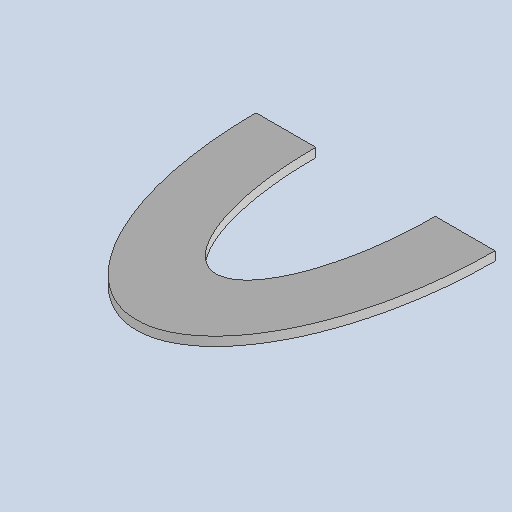
# Autodesk Inventor part: MSC 082 pillar 2
Saved by Autodesk Inventor 2025 (Build 290162010, 162A)
## iProperties
Created: 2024-06-25
Part Number: MSC 082 pillar 2
Material: Stainless Steel
Document SubType Name: Sheet Metal
Designer: admin
Density: 8 g/cm^3
Sheet Metal Rule: AISI304 3mm Die 32
Appearance: Default
Stock Number: Зап. часть
Mass: 80.4248 g
Surface Area: 77.6704 cm^2
Volume: 10.0531 cm^3
Flat Pattern Width: 8 cm
Flat Pattern Length: 8 cm
Flat Pattern Area: 64 cm^2
Sheet Metal Width: 80,000 mm
Sheet Metal Length: 80,000 mm
Sheet Metal Area: 6400,000 mm^2
Author: admin
Autodesk Inventor part; units mm, degrees
ref_plane "YZ Plane" through (0, 0, 0) normal (1, 0, 0) x (0, 1, 0)
ref_plane "XZ Plane" through (0, 0, 0) normal (0, 1, 0) x (-1, 0, 0)
ref_plane "XY Plane" through (0, 0, 0) normal (0, 0, 1) x (1, 0, 0)
sketch "Sketch1" plane through (0, 0, 0) normal (0, 0, 1) x (1, 0, 0)
  ellipse E0 centre (0, 0) end of major axis (0, -80) minor radius 40
  ellipse E1 centre (0, 0) end of major axis (0, -53.3333) minor radius 20
  line L0 (40, 0) -> (-40, 0)
  point P0 (-20, 0)
  point P1 (20, 0)
  dimension "d73" = 80
  dimension "d74" = 40
  dimension "d75" = 20
  dimension "d76" = 53.3333
extrude "Plate1" add sketch "Sketch1" along normal blind 3 contours E0 L0 E1 picked at (-33.0642, -5.3304)
equation "\"d75\" = 0.5 * d74"
equation "\"d76\" = 0.666667 * d73"
equation "\"d6\" = Thickness"
equation "\"BendReliefWidth\" = Thickness"
equation "\"BendReliefDepth\" = 0.5 * Thickness"
equation "\"CornerReliefSize\" = 4 * Thickness"
equation "\"MinimumRemnant\" = 2 * Thickness"
equation "\"TransitionRadius\" = BendRadius"
equation "\"JacobiRadiusSize\" = BendRadius"
equation "\"GapSize\" = Thickness"
equation "\"Thickness\" = 3"
equation "\"BendRadius\" = 5"
body "Solid1"
